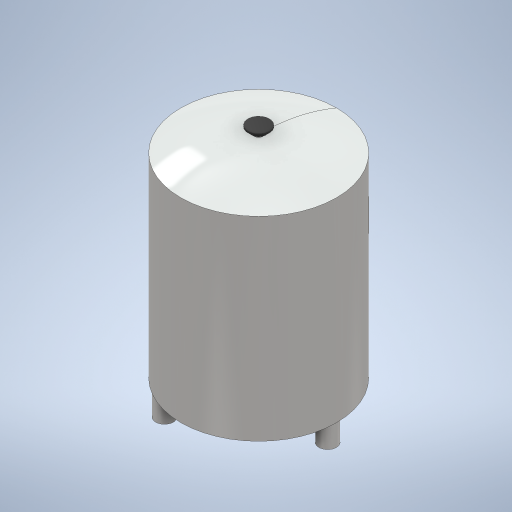
# Autodesk Inventor part: LauteringTun
Saved by Autodesk Inventor 2024 (Build 280153000, 153)
## iProperties
Created: 2025-09-20
Part Number: LauteringTun
Material: Generic
Document SubType Name: Modeling
Designer: Emil
Density: 1 g/cm^3
Appearance: Default
Author: Emil
Autodesk Inventor part; units mm, degrees
sketch "Sketch1" plane through (0, 0, 0) normal (0, 1, 0) x (-1, 0, 0)
  circle A0 centre (0, 0) radius 145
  circle A1 centre (0, 0) radius 120
  dimension "d0" = 290
  dimension "d1" = 240
  constraints: 2 centre point, 2 coincident
  measures "d0" diameter of A0
  measures "d1" diameter of A1
extrude "Extrusion1" add sketch "Sketch1" along normal blind 360
sketch "Sketch2" plane through (0, 0, 0) normal (0, -1, 0) x (1, 0, 0)
  circle A0 centre (0, 0) radius 145
  constraints: 1 centre point, 1 coincident
extrude "Extrusion2" add sketch "Sketch2" along normal blind 3
sketch "Sketch3" plane through (0, -3, 0) normal (0, -1, 0) x (1, 0, 0)
  circle A0 centre (0, 0) radius 145 projected
  circle A1 centre (128.5, 0) radius 16.5
  circle A2 centre (0, 0) radius 145 projected
  dimension "d6" = 33
  constraints: 1 centre point, 1 tangent
  measures "d6" diameter of A1
extrude "Extrusion3" add sketch "Sketch3" along normal blind 40 contours A1
pattern_circular "Circular Pattern1" count 3 over 360 about axis through (0, -10, 0) along (0, 1, 0) of "Extrusion3"
sketch "Sketch4" plane through (0, 0, 0) normal (1, 0, 0) x (0, 1, 0)
  line L0 (360, -145) -> (360, 145) projected
  line L1 (360, 0) -> (390, 0)
  line L2 (360, -145) -> (360, 0)
  spline S0 degree 2 poles (360, -145) (390, -72.5) (390, 0) knots 0 0 0 0.5 0.5 0.5
  line L3 (390, -28.8222) -> (390, 28.8222) construction
  arc A0 (389.2438, -23.008) -> (389.2438, 23.008) centre (39.5833, 0) ccw construction
  line L4 (-131.127, 0) -> (485.762, 0) projected
  point P0 (0, 0)
  dimension "d13" = 30
  constraints: 6 end point, 3 midpoint, 1 centre point, 1 collinear, 1 horizontal, 1 point on circle, 1 vertical, 3 other
  measures "d13" distance of L1.end L1.start
revolve "Revolution1" add sketch "Sketch4" angle 360 about axis through (0, -10, 0) along (0, 1, 0)
ref_plane "Work Plane2" through (0, 390, 0) normal (0, -1, 0) x (1, 0, 0)
sketch "Sketch5" plane through (0, 390, 0) normal (0, -1, 0) x (1, 0, 0)
  point P0 (0, 0)
sketch "Sketch6" plane through (0, 390, 0) normal (0, -1, 0) x (1, 0, 0)
  circle A0 centre (0, 0) radius 7.5
  dimension "d15" = 15
  constraints: 1 centre point, 1 coincident
  measures "d15" diameter of A0
extrude "Extrusion4" add sketch "Sketch6" against normal blind 5
sketch "Sketch7" plane through (0, 395, 0) normal (0, 1, 0) x (1, 0, 0)
  circle A0 centre (0, 0) radius 7.5 projected
  circle A1 centre (0, 0) radius 20
  dimension "d18" = 40
  constraints: 1 centre point, 1 coincident
  measures "d18" diameter of A1
extrude "Extrusion5" add sketch "Sketch7" along normal blind 10 contours A0 | A1
chamfer "Chamfer1" distance 7 angle 45 1 edges at (-20, 395, 0)
ref_plane "Work Plane3" through (-145, 0, 0) normal (1, 0, 0) x (0, 1, 0)
sketch "Sketch8" plane through (-145, 0, 0) normal (1, 0, 0) x (0, 1, 0)
  line L0 (0, 0) -> (40, 0) construction
  circle A0 centre (40, 0) radius 10
  dimension "d24" = 40
  dimension "d25" = 20
  constraints: 2 end point, 1 centre point, 1 coincident, 1 horizontal
  measures "d24" distance of L0.start L0.end
  measures "d25" diameter of A0
extrude "Extrusion6" add sketch "Sketch8" against normal blind 30
ref_plane "Work Plane4" through (-145, 40, 10) normal (0, 0, 1) x (1, 0, 0)
sketch "Sketch11" plane through (-145, 40, 10) normal (0, 0, 1) x (1, 0, 0)
  circle A0 centre (-20, 0) radius 10
  line L0 (0, 10) -> (-30, 10) projected
  line L1 (-30, 10) -> (-30, -10) projected
  point P0 (145, -40)
  constraints: 2 tangent, 1 centre point
extrude "Extrusion8" add sketch "Sketch11" against normal blind 60 contours A0
ref_plane "Work Plane5" through (0, 0, -145) normal (0, 0, 1) x (1, 0, 0)
sketch "Sketch12" plane through (0, 0, -145) normal (0, 0, 1) x (1, 0, 0)
  line L0 (-40, 167) -> (40, 167)
  line L1 (40, 167) -> (40, 227)
  line L2 (40, 227) -> (-40, 227)
  line L3 (-40, 227) -> (-40, 167)
  line L4 (-40, 167) -> (40, 227) construction
  line L5 (40, 167) -> (-40, 227) construction
  line L6 (-72.5, -3) -> (145, -3) projected
  point P0 (0, 0)
  point P1 (0, 197)
  dimension "d33" = 80
  dimension "d34" = 60
  dimension "d35" = 200
  constraints: 12 end point, 2 midpoint, 2 parallel, 1 horizontal, 1 perpendicular
  measures "d33" distance of L2.end L1.end
  measures "d34" distance of L1.end L0.end
  measures "d35" distance from line of L6 point (0, 197)
extrude "Extrusion9" add sketch "Sketch12" along normal mid plane 40
body "Solid1"
